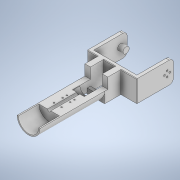
# Autodesk Inventor part: Tilt_Bracket_Output_2
Saved by Autodesk Inventor 2022 (Build 260153000, 153)
## iProperties
Created: 2022-02-26
Part Number: Tilt_Bracket_Output_2
Material: Generic
Document SubType Name: Modeling
Designer: Mlees
Density: 1 g/cm^3
Appearance: Default
Author: Mlees
Autodesk Inventor part; units mm, degrees
ref_plane "YZ Plane" through (0, 0, 0) normal (1, 0, 0) x (0, 1, 0)
ref_plane "XZ Plane" through (0, 0, 0) normal (0, 1, 0) x (-1, 0, 0)
ref_plane "XY Plane" through (0, 0, 0) normal (0, 0, 1) x (1, 0, 0)
sketch "Sketch1" plane through (0, 0, 0) normal (0, 1, 0) x (-1, 0, 0)
  line L0 (0, 0) -> (0, 62)
  line L1 (0, 62) -> (80, 62)
  line L2 (80, 62) -> (80, 0)
  line L3 (86, 0) -> (86, 68)
  line L4 (86, 68) -> (-6, 68)
  line L5 (-6, 68) -> (-6, 0)
  line L6 (80, 0) -> (86, 0)
  line L7 (-6, 0) -> (0, 0)
  dimension "d0" = 62
  dimension "d1" = 80
  dimension "d2" = 6
  dimension "d5" = 62
  constraints: 16 end point, 2 horizontal, 2 perpendicular, 1 collinear, 1 vertical, 2 other
  measures "d0" distance of L0.start L0.end
  measures "d1" distance of L0.end L1.end
  measures "d2" distance between parallel lines of L2 L3
  measures "d5" distance of L1.end L2.end
extrude "Extrusion1" add sketch "Sketch1" along normal blind 40
sketch "Sketch2" plane through (6, 0, 68) normal (1, 0, 0) x (0, 0, -1)
  line L0 (68, 0) -> (68, 40) projected
  circle A0 centre (56, 25) radius 1.5
  circle A1 centre (51, 20) radius 1.5
  circle A2 centre (56, 15) radius 1.5
  circle A3 centre (61, 20) radius 1.5
  point P0 (56, 20)
  dimension "d9" = 3
  dimension "d12" = 360
  constraints: 4 centre point, 9 other
  measures "d9" diameter of A0
extrude "Extrusion2" cut sketch "Sketch2" against normal up to surface (6 mm away)
sketch "Sketch3" plane through (-80, 0, 62) normal (1, 0, 0) x (0, 0, -1)
  line L0 (62, 0) -> (62, 40) projected
  line L1 (62, 20) -> (58, 20)
  circle A0 centre (50, 20) radius 5.75
  dimension "d16" = 4
  dimension "d18" = 11.5
  constraints: 2 end point, 1 centre point, 1 horizontal, 1 midpoint
  measures "d16" distance of L1.start L1.end
  measures "d18" diameter of A0
extrude "Extrusion3" add sketch "Sketch3" along normal blind 10
fillet "Fillet1" radius 8 4 edges at (3, 40, 0) (3, 0, 0) (-83, 0, 0) (-83, 40, 0)
sketch "Sketch4" plane through (-86, 0, 68) normal (0, 0, 1) x (1, 0, 0)
  line L0 (41, 0) -> (41, 20)
  line L1 (30, 0) -> (30, 40)
  line L2 (86, 40) -> (6, 40) projected
  line L3 (52, 0) -> (52, 40)
  line L4 (25, 0) -> (25, 40)
  line L5 (57, 0) -> (57, 40)
  line L6 (25, 40) -> (30, 40)
  line L7 (52, 40) -> (57, 40)
  line L8 (52, 0) -> (57, 0)
  line L9 (86, 0) -> (6, 0) projected
  line L10 (30, 0) -> (25, 0)
  dimension "d22" = 11
  dimension "d23" = 11
  dimension "d24" = 5
  dimension "d25" = 5
  constraints: 18 end point, 4 collinear, 2 parallel, 2 point on line, 1 perpendicular, 1 vertical
  measures "d22" distance of L0.start L3.start
  measures "d23" distance of L0.start L1.start
  measures "d24" distance between parallel lines of L1 L4
  measures "d25" distance between parallel lines of L3 L5
extrude "Extrusion4" add sketch "Sketch4" along normal blind 24 contours L9 L4 L2 L1 | L2 L5 L8 L3
sketch "Sketch5" plane through (-86, 0, 92) normal (0, 0, 1) x (1, 0, 0)
  line L0 (25, 0) -> (25, 40) projected
  line L1 (57, 0) -> (57, 40) projected
  line L2 (25, 0) -> (57, 0)
  line L3 (57, 0) -> (57, 40)
  line L4 (52, 0) -> (52, 40) projected
  line L5 (57, 40) -> (52, 40)
  line L6 (30, 0) -> (52, 0) projected
  line L7 (41, 3.3) -> (41, 9.3)
  line L8 (41, 9.3) -> (52, 9.3)
  line L9 (41, 9.3) -> (30, 9.3)
  line L10 (52, 9.3) -> (52, 40)
  line L11 (86, 40) -> (6, 40) projected
  line L12 (30, 40) -> (30, 0) projected
  line L13 (30, 9.3) -> (30, 40)
  line L14 (30, 40) -> (25, 40)
  line L15 (25, 40) -> (25, 0)
  line L16 (86, 0) -> (6, 0) projected
  dimension "d29" = 6
  constraints: 20 end point, 6 perpendicular, 2 collinear, 2 point on line
  measures "d29" distance of L7.start L7.end
extrude "Extrusion5" add sketch "Sketch5" along normal blind 6 contours L0 L11 L12 L2 | L12 L9 L8 L4 L2 | L4 L5 L1 L2
sketch "Sketch6" plane through (-86, 0, 98) normal (0, 0, 1) x (1, 0, 0)
  line L0 (25, 0) -> (25, 40) projected
  line L1 (25, 40) -> (25, 0)
  line L2 (57, 40) -> (57, 0) projected
  line L3 (25, 0) -> (57, 0)
  line L4 (57, 0) -> (57, 40)
  line L5 (52, 0) -> (52, 40) projected
  line L6 (57, 40) -> (52, 40)
  line L7 (30, 40) -> (25, 40) projected
  line L8 (25, 40) -> (30, 40)
  line L9 (30, 0) -> (52, 0) projected
  line L10 (30, 40) -> (30, 0)
  line L11 (30, 0) -> (52, 0)
  line L12 (52, 40) -> (52, 9.3) projected
  line L13 (52, 40) -> (52, 0)
  line L14 (25, 0) -> (57, 0) projected
  point P0 (86, 0)
  constraints: 16 end point, 6 perpendicular, 2 collinear
extrude "Extrusion6" add sketch "Sketch6" along normal blind 13.8
sketch "Sketch8" plane through (-86, 0, 111.8) normal (0, 0, 1) x (1, 0, 0)
  line L0 (52, 9.3) -> (30, 9.3) projected
  arc A0 (30.0455, 19.3) -> (51.9545, 19.3) centre (41, 20.3) ccw
  line L1 (51.9545, 19.3) -> (52, 19.3)
  line L2 (52, 0) -> (52, 40) projected
  line L3 (30, 40) -> (52, 40) projected
  line L4 (52, 19.3) -> (52, 40)
  line L5 (57, 40) -> (52, 40) projected
  line L6 (52, 40) -> (57, 40)
  line L7 (57, 40) -> (57, 6.3)
  line L8 (57, 40) -> (57, 0) projected
  line L9 (57, 6.3) -> (25, 6.3)
  line L10 (25, 0) -> (25, 40) projected
  line L11 (0, 40) -> (25, 40) projected
  line L12 (25, 6.3) -> (25, 40)
  line L13 (25, 40) -> (30, 40)
  line L14 (30, 40) -> (30, 19.3)
  line L15 (30, 40) -> (30, 0) projected
  line L16 (30, 19.3) -> (30.0455, 19.3)
  point P0 (86, 0)
  dimension "d37" = 33.7
  dimension "d38" = 11
  constraints: 18 end point, 6 point on line, 3 perpendicular, 2 point on circle, 2 vertical, 1 centre point, 1 horizontal, 1 tangent
  measures "d37" distance of L5.start L7.end
  measures "d38" radius of A0
extrude "Extrusion7" add sketch "Sketch8" along normal blind 13.8 contours L2 L9 L15 L0 | L0 A0 L1 L2 | L2 L5 L7 L9 | L0 L15 L16 A0 | L15 L9 L10 L13 L14
sketch "Sketch9" plane through (-86, 0, 125.6) normal (0, 0, 1) x (1, 0, 0)
  line L0 (25, 6.3) -> (57, 6.3) projected
  arc A0 (30.0455, 19.3) -> (51.9545, 19.3) centre (41, 20.3) ccw projected
  arc A1 (38, 20.3) -> (44, 20.3) centre (41, 20.3) ccw
  line L1 (25, 40) -> (25, 6.3) projected
  line L2 (25, 6.3) -> (25, 40)
  line L3 (57, 6.3) -> (57, 40) projected
  line L4 (25, 40) -> (57, 40)
  line L5 (38, 20.3) -> (30, 20.3)
  line L6 (30, 19.3) -> (30, 40) projected
  line L7 (44, 20.3) -> (52, 20.3)
  line L8 (52, 40) -> (52, 20.3)
  line L9 (52, 40) -> (57, 40)
  line L10 (57, 40) -> (57, 6.3)
  line L11 (57, 6.3) -> (25, 6.3)
  point P0 (86, 0)
  dimension "d41" = 6
  constraints: 16 end point, 3 collinear, 3 perpendicular, 2 point on circle, 2 point on line, 1 centre point, 1 coincident, 1 horizontal
  measures "d41" diameter of A1
extrude "Extrusion8" add sketch "Sketch9" along normal blind 50 contours L1 L4 L6 L5 A1 L7 L8 L3 L0
sketch "Sketch10" plane through (0, 40, 0) normal (0, 1, 0) x (1, 0, 0)
  line L0 (-34, -98) -> (-56, -98) projected
  line L1 (-56, -98) -> (-34, -98)
  line L2 (-34, -175.6) -> (-56, -175.6)
  line L3 (-29, -68) -> (-29, -175.6) projected
  line L4 (-29, -175.6) -> (-34, -175.6)
  line L5 (-34, -175.6) -> (-34, -98)
  line L6 (-34, -98) -> (-29, -98)
  line L7 (-29, -98) -> (-29, -175.6)
  line L8 (-61, -175.6) -> (-29, -175.6) projected
  line L9 (-61, -175.6) -> (-56, -175.6)
  line L10 (-56, -98) -> (-61, -98)
  line L11 (-61, -98) -> (-61, -175.6)
  point P0 (0, 0)
  point P1 (-29, -98)
  constraints: 18 end point, 4 parallel, 3 horizontal, 1 perpendicular
extrude "Extrusion9" cut sketch "Sketch10" against normal up to surface (19.7 mm away)
sketch "Sketch11" plane through (-86, 0, 175.6) normal (0, 0, 1) x (1, 0, 0)
  arc A0 (38, 20.3) -> (44, 20.3) centre (41, 20.3) ccw projected
  line L0 (52, 20.3) -> (44, 20.3) projected
  arc A1 (19.7397, 20.3) -> (62.2603, 20.3) centre (41, 20.3) ccw
  arc A2 (38, 20.3) -> (44, 20.3) centre (41, 20.3) ccw
  line L1 (19.7397, 20.3) -> (38, 20.3)
  line L2 (44, 20.3) -> (62.2603, 20.3)
  point P0 (86, 0)
  constraints: 4 end point, 4 point on circle, 2 centre point, 2 coincident, 2 horizontal
extrude "Extrusion10" add sketch "Sketch11" along normal blind 36
sketch "Sketch12" plane through (-86, 0, 211.6) normal (0, 0, 1) x (1, 0, 0)
  arc A0 (38, 20.3) -> (44, 20.3) centre (41, 20.3) ccw projected
  circle A1 centre (41, 20.3) radius 19
  point P0 (86, 0)
  dimension "d49" = 38
  constraints: 1 centre point, 1 coincident
  measures "d49" diameter of A1
extrude "Extrusion11" cut sketch "Sketch12" against normal blind 32
sketch "Sketch13" plane through (-86, 0, 211.6) normal (0, 0, 1) x (1, 0, 0)
  line L0 (62.2603, 20.3) -> (57, 20.3) projected
  arc A0 (19.7397, 20.3) -> (62.2603, 20.3) centre (41, 20.3) ccw
  line L1 (22, 20.3) -> (38, 20.3) projected
  arc A1 (22, 20.3) -> (60, 20.3) centre (41, 20.3) ccw projected
  arc A2 (22, 20.3) -> (60, 20.3) centre (41, 20.3) ccw
  line L2 (19.7397, 20.3) -> (22, 20.3)
  line L3 (62.2603, 20.3) -> (60, 20.3)
  point P0 (86, 0)
  constraints: 4 end point, 4 point on circle, 2 centre point, 1 collinear, 1 horizontal
extrude "Extrusion12" add sketch "Sketch13" along normal blind 6.2
fillet "Fillet3" radius 1 5 edges at (-86, 20, 68) (-45, 40, 68) (-11.5, 40, 68) (-73.5, 40, 68) (6, 20, 68)
sketch "Sketch20" plane through (-29, 0, 111.8) normal (1, 0, 0) x (0, 0, -1)
  line L0 (0, 6.3) -> (-63.8, 6.3) projected
  line L1 (0, 6.3) -> (0, 0) projected
  line L2 (-63.8, 6.3) -> (0, 6.3)
  line L3 (0, 6.3) -> (0, 0)
  line L4 (0, 0) -> (-63.8, 0)
  line L5 (-63.8, 0) -> (-63.8, 6.3)
  point P0 (111.8, 0)
  constraints: 8 end point, 2 parallel, 1 horizontal, 1 perpendicular
extrude "Extrusion19" add sketch "Sketch20" against normal up to surface (5 mm away)
sketch "Sketch21" plane through (-61, 0, 68) normal (-1, 0, 0) x (0, 0, 1)
  line L0 (43.8, 6.3) -> (107.6, 6.3) projected
  line L1 (0, 0) -> (107.6, 0) projected
  line L2 (43.8, 6.3) -> (107.6, 6.3)
  line L3 (107.6, 6.3) -> (107.6, 0)
  line L4 (107.6, 0) -> (43.8, 0)
  line L5 (43.8, 0) -> (43.8, 6.3)
  point P0 (-68, 0)
  point P1 (107.6, 6.3)
  point P2 (43.8, 0)
  constraints: 8 end point, 2 parallel, 1 horizontal, 1 perpendicular
extrude "Extrusion20" add sketch "Sketch21" against normal up to surface (5 mm away)
sketch "Sketch22" plane through (-61, 20.3, 98) normal (-1, 0, 0) x (0, 0, 1)
  line L0 (-31, 19.7) -> (0, 19.7) projected
  line L1 (-31, 19.7) -> (0, 19.7)
  line L2 (0, 0) -> (27.6, 0) projected
  line L3 (0, 19.7) -> (0, 0)
  line L4 (77.6, 0) -> (119.8, 0) projected
  line L5 (0, 0) -> (77.6, 0)
  line L6 (-30, -20.3) -> (77.6, -20.3) projected
  line L7 (77.6, 0) -> (77.6, -20.3)
  line L8 (-31, 19.7) -> (-31, -20.3) projected
  line L9 (77.6, -20.3) -> (-31, -20.3)
  line L10 (-31, -20.3) -> (-31, 19.7)
  point P0 (-98, -20.3)
  point P1 (-30, -20.3)
  constraints: 12 end point, 4 perpendicular, 1 collinear, 1 horizontal
extrude "Extrusion21" add sketch "Sketch22" along normal up to surface (5.2603 mm away)
sketch "Sketch23" plane through (-29, 20.3, 98) normal (1, 0, 0) x (0, 0, -1)
  line L0 (31, 19.7) -> (0, 19.7) projected
  line L1 (0, 19.7) -> (0, 0) projected
  line L2 (0, 19.7) -> (0, 0)
  line L3 (0, 0) -> (-77.6, 0) projected
  line L4 (0, 0) -> (-77.6, 0)
  line L5 (-77.6, -20.3) -> (-77.6, -18.1934) projected
  line L6 (-77.6, 0) -> (-77.6, -20.3)
  line L7 (31, 19.7) -> (31, -20.3) projected
  line L8 (-77.6, -20.3) -> (31, -20.3)
  line L9 (31, -20.3) -> (31, 19.7)
  line L10 (31, 19.7) -> (0, 19.7)
  point P0 (98, -20.3)
  constraints: 12 end point, 3 collinear, 3 perpendicular
extrude "Extrusion22" add sketch "Sketch23" along normal up to surface (5.2603 mm away)
sketch "Sketch24" plane through (-34, 0, 175.6) normal (0, 0, 1) x (1, 0, 0)
  line L0 (0, 2.1066) -> (0, 0) projected
  line L1 (0, 20.3) -> (10.2603, 20.3) projected
  arc A0 (0, 2.1066) -> (10.2603, 20.3) centre (-11, 20.3) ccw
  line L2 (-32.2603, 20.3) -> (-32.2603, 0) projected
  line L3 (-22, 0) -> (-22, 2.1066) projected
  arc A1 (-32.2603, 20.3) -> (-22, 2.1066) centre (-11, 20.3) ccw
  line L4 (-32.2603, 20.3) -> (-32.2603, 0)
  line L5 (34, 0) -> (-46, 0) projected
  line L6 (-22, 0) -> (-32.2603, 0)
  line L7 (-22, 0) -> (-22, 2.1066)
  line L8 (0, 0) -> (0, 2.1066)
  line L9 (10.2603, 39) -> (10.2603, 0) projected
  line L10 (10.2603, 0) -> (0, 0)
  arc A2 (0, 2.1066) -> (10.2603, 20.3) centre (-11, 20.3) ccw projected
  line L11 (10.2603, 0) -> (10.2603, 20.3)
  constraints: 12 end point, 4 perpendicular, 4 point on circle, 2 centre point, 2 equal length, 2 tangent
extrude "Extrusion23" cut sketch "Sketch24" against normal up to surface (77.6 mm away)
sketch "Sketch25" plane through (-56, 6.3, 111.8) normal (0, -1, 0) x (1, 0, 0)
  line L0 (0, 0) -> (22, 0) projected
  line L1 (-5, 63.8) -> (27, 63.8) projected
  line L2 (0, 63.8) -> (0, 0) projected
  line L3 (0, 63.8) -> (11, 63.8)
  line L4 (0, 63.8) -> (4, 63.8)
  line L5 (0.0455, 0) -> (21.9545, 0) projected
  line L6 (11, 0) -> (11, 63.8)
  circle A0 centre (4, 28) radius 1.25
  circle A1 centre (4, 35.8) radius 1.25
  circle A2 centre (4, 51.8) radius 1.25
  circle A3 centre (18, 28) radius 1.25
  circle A4 centre (18, 35.8) radius 1.25
  circle A5 centre (18, 51.8) radius 1.25
  point P0 (56, -111.8)
  point P1 (22, 63.8)
  dimension "d86" = 4
  dimension "d90" = 2.5
  constraints: 6 centre point, 6 end point, 3 symmetric about line, 2 midpoint, 1 collinear, 1 perpendicular, 1 point on line, 3 other
  measures "d86" distance of L2.start L4.end
  measures "d90" diameter of A0
extrude "Extrusion24" cut sketch "Sketch25" against normal through all contours A0 | A1 | A2 | A3 | A4 | A5
sketch "Sketch26" plane through (-23.7397, 0, 68) normal (1, 0, 0) x (0, 0, -1)
  line L0 (-30, 20.3) -> (-57.6, 20.3) projected
  line L1 (1, 40) -> (-30, 40) projected
  line L2 (-30, 20.3) -> (-24, 20.3)
  line L3 (-24, 20.3) -> (-24, 40)
  line L4 (-24, 40) -> (-30, 40)
  line L5 (-30, 40) -> (-30, 20.3)
  point P0 (68, 0)
  dimension "d91" = 6
  constraints: 8 end point, 2 parallel, 1 horizontal, 1 perpendicular, 1 point on line
  measures "d91" distance of L4.end L3.end
extrude "Extrusion25" cut sketch "Sketch26" against normal up to surface (42.5206 mm away)
sketch "Sketch27" plane through (-70, 20, 12) normal (1, 0, 0) x (0, 0, -1)
  line L0 (0, 0) -> (0, -5.75)
  circle A0 centre (0, 0) radius 5.75 projected
  point P0 (12, -20)
  constraints: 2 end point, 1 vertical, 1 vertical alignment, 1 other
ref_plane "Work Plane2" through (-70, 14.25, 12) normal (0, -1, 0) x (1, 0, 0)
sketch "Sketch28" plane through (-70, 14.25, 12) normal (0, -1, 0) x (1, 0, 0)
  line L0 (0, -5.75) -> (0, 5.75) projected
  circle A0 centre (-3, 0) radius 2.2
  point P0 (70, -12)
  dimension "d95" = 4.4
  constraints: 1 centre point
  measures "d95" diameter of A0
extrude "Extrusion26" cut sketch "Sketch28" against normal blind 4.2
body "Solid1"
